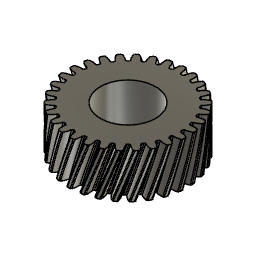
Helical Gear (Autodesk Fusion 360 design; units mm, degrees)
Autodesk Fusion 360 part; units mm, degrees
sketch "Base" plane through (0, 0, 0) normal (0, 0, 1) x (1, 0, 0)
  line L0 (0, 0) -> (8, 0) construction
  arc A0 (0.3264, 4.7068) -> (0.2135, 5.3108) centre (-1.2536, 4.724) ccw
  arc A1 (0.4834, 4.5997) -> (0.4173, 4.6061) centre (0, 0) ccw
  arc A2 (0.1229, 5.3736) -> (0, 5.375) centre (0, 0) ccw
  arc A3 (0.2135, 5.3108) -> (0.1229, 5.3736) centre (0.1206, 5.2736) ccw
  arc A4 (0.3264, 4.7068) -> (0.4173, 4.6061) centre (0.4264, 4.7057) ccw
  arc A5 (0, 5.375) -> (-0.1229, 5.3736) centre (0, 0) ccw
  arc A6 (-0.1229, 5.3736) -> (-0.2135, 5.3108) centre (-0.1206, 5.2736) ccw
  arc A7 (-0.2135, 5.3108) -> (-0.3264, 4.7068) centre (1.2536, 4.724) ccw
  arc A8 (-0.4173, 4.6061) -> (-0.3264, 4.7068) centre (-0.4264, 4.7057) ccw
  arc A9 (-0.4173, 4.6061) -> (-0.4834, 4.5997) centre (0, 0) ccw
  arc A10 (-1.1175, 5.2575) -> (-1.2375, 5.2306) centre (0, 0) ccw
  arc A11 (-0.997, 5.2817) -> (-1.1175, 5.2575) centre (0, 0) ccw
  arc A12 (-1.3659, 4.4187) -> (-1.2978, 4.5361) centre (-1.3954, 4.5142) ccw
  arc A13 (-0.6594, 4.6718) -> (-0.5494, 4.5922) centre (-0.5613, 4.6915) ccw
  arc A14 (-0.8954, 5.2391) -> (-0.997, 5.2817) centre (-0.9785, 5.1835) ccw
  arc A15 (-0.4834, 4.5997) -> (-0.5494, 4.5922) centre (0, 0) ccw
  arc A16 (-1.2375, 5.2306) -> (-1.313, 5.1503) centre (-1.2144, 5.1333) ccw
  arc A17 (-1.3659, 4.4187) -> (-1.4292, 4.3986) centre (0, 0) ccw
  arc A18 (-1.313, 5.1503) -> (-1.2978, 4.5361) centre (0.244, 4.8814) ccw
  arc A19 (-0.6594, 4.6718) -> (-0.8954, 5.2391) centre (-2.2084, 4.3601) ccw
  arc A20 (-2.1862, 4.9103) -> (-2.2979, 4.859) centre (0, 0) ccw
  arc A21 (-2.0734, 4.959) -> (-2.1862, 4.9103) centre (0, 0) ccw
  arc A22 (-2.2548, 4.0382) -> (-2.2126, 4.1671) centre (-2.3035, 4.1255) ccw
  arc A23 (-1.6163, 4.4326) -> (-1.4922, 4.3777) centre (-1.5245, 4.4723) ccw
  arc A24 (-1.9651, 4.9384) -> (-2.0734, 4.959) centre (-2.0348, 4.8668) ccw
  arc A25 (-1.4292, 4.3986) -> (-1.4922, 4.3777) centre (0, 0) ccw
  arc A26 (-2.2979, 4.859) -> (-2.3551, 4.7648) centre (-2.2552, 4.7686) ccw
  arc A27 (-2.2548, 4.0382) -> (-2.3125, 4.0054) centre (0, 0) ccw
  arc A28 (-2.3551, 4.7648) -> (-2.2126, 4.1671) centre (-0.7762, 4.8254) ccw
  arc A29 (-1.6163, 4.4326) -> (-1.9651, 4.9384) centre (-3.0666, 3.8057) ccw
  arc A30 (-3.1593, 4.3485) -> (-3.258, 4.2751) centre (0, 0) ccw
  arc A31 (-3.0591, 4.4196) -> (-3.1593, 4.3485) centre (0, 0) ccw
  arc A32 (-3.0451, 3.4811) -> (-3.0306, 3.616) centre (-3.1109, 3.5564) ccw
  arc A33 (-2.5025, 3.9997) -> (-2.3698, 3.9718) centre (-2.421, 4.0576) ccw
  arc A34 (-2.9489, 4.422) -> (-3.0591, 4.4196) centre (-3.0022, 4.3373) ccw
  arc A35 (-2.3125, 4.0054) -> (-2.3698, 3.9718) centre (0, 0) ccw
  arc A36 (-3.258, 4.2751) -> (-3.2943, 4.171) centre (-3.1973, 4.1956) ccw
  arc A37 (-3.0451, 3.4811) -> (-3.0947, 3.437) centre (0, 0) ccw
  arc A38 (-3.2943, 4.171) -> (-3.0306, 3.616) centre (-1.7625, 4.5586) ccw
  arc A39 (-2.5025, 3.9997) -> (-2.9489, 4.422) centre (-3.7908, 3.0849) ccw
  arc A40 (-3.9944, 3.5966) -> (-4.0756, 3.5043) centre (0, 0) ccw
  arc A41 (-3.9111, 3.687) -> (-3.9944, 3.5966) centre (0, 0) ccw
  arc A42 (-3.7023, 2.772) -> (-3.7162, 2.9069) centre (-3.7823, 2.8319) ccw
  arc A43 (-3.2794, 3.392) -> (-3.1438, 3.3923) centre (-3.2117, 3.4656) ccw
  arc A44 (-3.8038, 3.7122) -> (-3.9111, 3.687) centre (-3.8384, 3.6184) ccw
  arc A45 (-3.0947, 3.437) -> (-3.1438, 3.3923) centre (0, 0) ccw
  arc A46 (-4.0756, 3.5043) -> (-4.0895, 3.395) centre (-3.9998, 3.4391) ccw
  arc A47 (-3.7023, 2.772) -> (-3.7417, 2.7185) centre (0, 0) ccw
  arc A48 (-4.0895, 3.395) -> (-3.7162, 2.9069) centre (-2.6718, 4.0925) ccw
  arc A49 (-3.2794, 3.392) -> (-3.8038, 3.7122) centre (-4.3494, 2.2294) ccw
  arc A50 (-4.6549, 2.6875) -> (-4.7151, 2.5804) centre (0, 0) ccw
  arc A51 (-4.5922, 2.7932) -> (-4.6549, 2.6875) centre (0, 0) ccw
  arc A52 (-4.1977, 1.9416) -> (-4.2394, 2.0708) centre (-4.2885, 1.9836) ccw
  arc A53 (-3.913, 2.6361) -> (-3.7804, 2.6645) centre (-3.8621, 2.7221) ccw
  arc A54 (-4.4925, 2.8402) -> (-4.5922, 2.7932) centre (-4.5068, 2.7413) ccw
  arc A55 (-3.7417, 2.7185) -> (-3.7804, 2.6645) centre (0, 0) ccw
  arc A56 (-4.7151, 2.5804) -> (-4.706, 2.4705) centre (-4.6274, 2.5324) ccw
  arc A57 (-4.1977, 1.9416) -> (-4.2251, 1.8812) centre (0, 0) ccw
  arc A58 (-4.706, 2.4705) -> (-4.2394, 2.0708) centre (-3.4643, 3.4476) ccw
  arc A59 (-3.913, 2.6361) -> (-4.4925, 2.8402) centre (-4.7179, 1.2763) ccw
  arc A60 (-5.1119, 1.661) -> (-5.1486, 1.5436) centre (0, 0) ccw
  arc A61 (-5.0726, 1.7774) -> (-5.1119, 1.661) centre (0, 0) ccw
  arc A62 (-4.5097, 1.0264) -> (-4.5773, 1.1441) centre (-4.6072, 1.0486) ccw
  arc A63 (-4.3756, 1.7649) -> (-4.2517, 1.8203) centre (-4.3437, 1.8597) ccw
  arc A64 (-4.9849, 1.8441) -> (-5.0726, 1.7774) centre (-4.9782, 1.7444) ccw
  arc A65 (-4.2251, 1.8812) -> (-4.2517, 1.8203) centre (0, 0) ccw
  arc A66 (-5.1486, 1.5436) -> (-5.1168, 1.4381) centre (-5.0528, 1.5149) ccw
  arc A67 (-4.5097, 1.0264) -> (-4.5239, 0.9616) centre (0, 0) ccw
  arc A68 (-5.1168, 1.4381) -> (-4.5773, 1.1441) centre (-4.1054, 2.652) ccw
  arc A69 (-4.3756, 1.7649) -> (-4.9849, 1.8441) centre (-4.8801, 0.2676) ccw
  arc A70 (-5.3456, 0.5618) -> (-5.357, 0.4395) centre (0, 0) ccw
  arc A71 (-5.3313, 0.6839) -> (-5.3456, 0.5618) centre (0, 0) ccw
  arc A72 (-4.6245, 0.0664) -> (-4.7151, 0.1674) centre (-4.7245, 0.0678) ccw
  arc A73 (-4.6469, 0.8166) -> (-4.5373, 0.8965) centre (-4.6354, 0.9159) ccw
  arc A74 (-5.2594, 0.7674) -> (-5.3313, 0.6839) centre (-5.2321, 0.6712) ccw
  arc A75 (-4.5239, 0.9616) -> (-4.5373, 0.8965) centre (0, 0) ccw
  arc A76 (-5.357, 0.4395) -> (-5.304, 0.3428) centre (-5.2573, 0.4313) ccw
  arc A77 (-4.6245, 0.0664) -> (-4.625, 0) centre (0, 0) ccw
  arc A78 (-5.304, 0.3428) -> (-4.7151, 0.1674) centre (-4.567, 1.7405) ccw
  arc A79 (-4.6469, 0.8166) -> (-5.2594, 0.7674) centre (-4.8291, -0.7529) ccw
  arc A80 (-5.3456, -0.5618) -> (-5.3313, -0.6839) centre (0, 0) ccw
  arc A81 (-5.357, -0.4395) -> (-5.3456, -0.5618) centre (0, 0) ccw
  arc A82 (-4.5373, -0.8965) -> (-4.6469, -0.8166) centre (-4.6354, -0.9159) ccw
  arc A83 (-4.7151, -0.1674) -> (-4.6245, -0.0664) centre (-4.7245, -0.0678) ccw
  arc A84 (-5.304, -0.3428) -> (-5.357, -0.4395) centre (-5.2573, -0.4313) ccw
  arc A85 (-4.625, 0) -> (-4.6245, -0.0664) centre (0, 0) ccw
  arc A86 (-5.3313, -0.6839) -> (-5.2594, -0.7674) centre (-5.2321, -0.6712) ccw
  arc A87 (-4.5373, -0.8965) -> (-4.5239, -0.9616) centre (0, 0) ccw
  arc A88 (-5.2594, -0.7674) -> (-4.6469, -0.8166) centre (-4.8291, 0.7529) ccw
  arc A89 (-4.7151, -0.1674) -> (-5.304, -0.3428) centre (-4.567, -1.7405) ccw
  arc A90 (-5.1119, -1.661) -> (-5.0726, -1.7774) centre (0, 0) ccw
  arc A91 (-5.1486, -1.5436) -> (-5.1119, -1.661) centre (0, 0) ccw
  arc A92 (-4.2517, -1.8203) -> (-4.3756, -1.7649) centre (-4.3437, -1.8597) ccw
  arc A93 (-4.5773, -1.1441) -> (-4.5097, -1.0264) centre (-4.6072, -1.0486) ccw
  arc A94 (-5.1168, -1.4381) -> (-5.1486, -1.5436) centre (-5.0528, -1.5149) ccw
  arc A95 (-4.5239, -0.9616) -> (-4.5097, -1.0264) centre (0, 0) ccw
  arc A96 (-5.0726, -1.7774) -> (-4.9849, -1.8441) centre (-4.9782, -1.7444) ccw
  arc A97 (-4.2517, -1.8203) -> (-4.2251, -1.8812) centre (0, 0) ccw
  arc A98 (-4.9849, -1.8441) -> (-4.3756, -1.7649) centre (-4.8801, -0.2676) ccw
  arc A99 (-4.5773, -1.1441) -> (-5.1168, -1.4381) centre (-4.1054, -2.652) ccw
  arc A100 (-4.6549, -2.6875) -> (-4.5922, -2.7932) centre (0, 0) ccw
  arc A101 (-4.7151, -2.5804) -> (-4.6549, -2.6875) centre (0, 0) ccw
  arc A102 (-3.7804, -2.6645) -> (-3.913, -2.6361) centre (-3.8621, -2.7221) ccw
  arc A103 (-4.2394, -2.0708) -> (-4.1977, -1.9416) centre (-4.2885, -1.9836) ccw
  arc A104 (-4.706, -2.4705) -> (-4.7151, -2.5804) centre (-4.6274, -2.5324) ccw
  arc A105 (-4.2251, -1.8812) -> (-4.1977, -1.9416) centre (0, 0) ccw
  arc A106 (-4.5922, -2.7932) -> (-4.4925, -2.8402) centre (-4.5068, -2.7413) ccw
  arc A107 (-3.7804, -2.6645) -> (-3.7417, -2.7185) centre (0, 0) ccw
  arc A108 (-4.4925, -2.8402) -> (-3.913, -2.6361) centre (-4.7179, -1.2763) ccw
  arc A109 (-4.2394, -2.0708) -> (-4.706, -2.4705) centre (-3.4643, -3.4476) ccw
  arc A110 (-3.9944, -3.5966) -> (-3.9111, -3.687) centre (0, 0) ccw
  arc A111 (-4.0756, -3.5043) -> (-3.9944, -3.5966) centre (0, 0) ccw
  arc A112 (-3.1438, -3.3923) -> (-3.2794, -3.392) centre (-3.2117, -3.4656) ccw
  arc A113 (-3.7162, -2.9069) -> (-3.7023, -2.772) centre (-3.7823, -2.8319) ccw
  arc A114 (-4.0895, -3.395) -> (-4.0756, -3.5043) centre (-3.9998, -3.4391) ccw
  arc A115 (-3.7417, -2.7185) -> (-3.7023, -2.772) centre (0, 0) ccw
  arc A116 (-3.9111, -3.687) -> (-3.8038, -3.7122) centre (-3.8384, -3.6184) ccw
  arc A117 (-3.1438, -3.3923) -> (-3.0947, -3.437) centre (0, 0) ccw
  arc A118 (-3.8038, -3.7122) -> (-3.2794, -3.392) centre (-4.3494, -2.2294) ccw
  arc A119 (-3.7162, -2.9069) -> (-4.0895, -3.395) centre (-2.6718, -4.0925) ccw
  arc A120 (-3.1593, -4.3485) -> (-3.0591, -4.4196) centre (0, 0) ccw
  arc A121 (-3.258, -4.2751) -> (-3.1593, -4.3485) centre (0, 0) ccw
  arc A122 (-2.3698, -3.9718) -> (-2.5025, -3.9997) centre (-2.421, -4.0576) ccw
  arc A123 (-3.0306, -3.616) -> (-3.0451, -3.4811) centre (-3.1109, -3.5564) ccw
  arc A124 (-3.2943, -4.171) -> (-3.258, -4.2751) centre (-3.1973, -4.1956) ccw
  arc A125 (-3.0947, -3.437) -> (-3.0451, -3.4811) centre (0, 0) ccw
  arc A126 (-3.0591, -4.4196) -> (-2.9489, -4.422) centre (-3.0022, -4.3373) ccw
  arc A127 (-2.3698, -3.9718) -> (-2.3125, -4.0054) centre (0, 0) ccw
  arc A128 (-2.9489, -4.422) -> (-2.5025, -3.9997) centre (-3.7908, -3.0849) ccw
  arc A129 (-3.0306, -3.616) -> (-3.2943, -4.171) centre (-1.7625, -4.5586) ccw
  arc A130 (-2.1862, -4.9103) -> (-2.0734, -4.959) centre (0, 0) ccw
  arc A131 (-2.2979, -4.859) -> (-2.1862, -4.9103) centre (0, 0) ccw
  arc A132 (-1.4922, -4.3777) -> (-1.6163, -4.4326) centre (-1.5245, -4.4723) ccw
  arc A133 (-2.2126, -4.1671) -> (-2.2548, -4.0382) centre (-2.3035, -4.1255) ccw
  arc A134 (-2.3551, -4.7648) -> (-2.2979, -4.859) centre (-2.2552, -4.7686) ccw
  arc A135 (-2.3125, -4.0054) -> (-2.2548, -4.0382) centre (0, 0) ccw
  arc A136 (-2.0734, -4.959) -> (-1.9651, -4.9384) centre (-2.0348, -4.8668) ccw
  arc A137 (-1.4922, -4.3777) -> (-1.4292, -4.3986) centre (0, 0) ccw
  arc A138 (-1.9651, -4.9384) -> (-1.6163, -4.4326) centre (-3.0666, -3.8057) ccw
  arc A139 (-2.2126, -4.1671) -> (-2.3551, -4.7648) centre (-0.7762, -4.8254) ccw
  arc A140 (-1.1175, -5.2575) -> (-0.997, -5.2817) centre (0, 0) ccw
  arc A141 (-1.2375, -5.2306) -> (-1.1175, -5.2575) centre (0, 0) ccw
  arc A142 (-0.5494, -4.5922) -> (-0.6594, -4.6718) centre (-0.5613, -4.6915) ccw
  arc A143 (-1.2978, -4.5361) -> (-1.3659, -4.4187) centre (-1.3954, -4.5142) ccw
  arc A144 (-1.313, -5.1503) -> (-1.2375, -5.2306) centre (-1.2144, -5.1333) ccw
  arc A145 (-1.4292, -4.3986) -> (-1.3659, -4.4187) centre (0, 0) ccw
  arc A146 (-0.997, -5.2817) -> (-0.8954, -5.2391) centre (-0.9785, -5.1835) ccw
  arc A147 (-0.5494, -4.5922) -> (-0.4834, -4.5997) centre (0, 0) ccw
  arc A148 (-0.8954, -5.2391) -> (-0.6594, -4.6718) centre (-2.2084, -4.3601) ccw
  arc A149 (-1.2978, -4.5361) -> (-1.313, -5.1503) centre (0.244, -4.8814) ccw
  arc A150 (0, -5.375) -> (0.1229, -5.3736) centre (0, 0) ccw
  arc A151 (-0.1229, -5.3736) -> (0, -5.375) centre (0, 0) ccw
  arc A152 (0.4173, -4.6061) -> (0.3264, -4.7068) centre (0.4264, -4.7057) ccw
  arc A153 (-0.3264, -4.7068) -> (-0.4173, -4.6061) centre (-0.4264, -4.7057) ccw
  arc A154 (-0.2135, -5.3108) -> (-0.1229, -5.3736) centre (-0.1206, -5.2736) ccw
  arc A155 (-0.4834, -4.5997) -> (-0.4173, -4.6061) centre (0, 0) ccw
  arc A156 (0.1229, -5.3736) -> (0.2135, -5.3108) centre (0.1206, -5.2736) ccw
  arc A157 (0.4173, -4.6061) -> (0.4834, -4.5997) centre (0, 0) ccw
  arc A158 (0.2135, -5.3108) -> (0.3264, -4.7068) centre (-1.2536, -4.724) ccw
  arc A159 (-0.3264, -4.7068) -> (-0.2135, -5.3108) centre (1.2536, -4.724) ccw
  arc A160 (1.1175, -5.2575) -> (1.2375, -5.2306) centre (0, 0) ccw
  arc A161 (0.997, -5.2817) -> (1.1175, -5.2575) centre (0, 0) ccw
  arc A162 (1.3659, -4.4187) -> (1.2978, -4.5361) centre (1.3954, -4.5142) ccw
  arc A163 (0.6594, -4.6718) -> (0.5494, -4.5922) centre (0.5613, -4.6915) ccw
  arc A164 (0.8954, -5.2391) -> (0.997, -5.2817) centre (0.9785, -5.1835) ccw
  arc A165 (0.4834, -4.5997) -> (0.5494, -4.5922) centre (0, 0) ccw
  arc A166 (1.2375, -5.2306) -> (1.313, -5.1503) centre (1.2144, -5.1333) ccw
  arc A167 (1.3659, -4.4187) -> (1.4292, -4.3986) centre (0, 0) ccw
  arc A168 (1.313, -5.1503) -> (1.2978, -4.5361) centre (-0.244, -4.8814) ccw
  arc A169 (0.6594, -4.6718) -> (0.8954, -5.2391) centre (2.2084, -4.3601) ccw
  arc A170 (2.1862, -4.9103) -> (2.2979, -4.859) centre (0, 0) ccw
  arc A171 (2.0734, -4.959) -> (2.1862, -4.9103) centre (0, 0) ccw
  arc A172 (2.2548, -4.0382) -> (2.2126, -4.1671) centre (2.3035, -4.1255) ccw
  arc A173 (1.6163, -4.4326) -> (1.4922, -4.3777) centre (1.5245, -4.4723) ccw
  arc A174 (1.9651, -4.9384) -> (2.0734, -4.959) centre (2.0348, -4.8668) ccw
  arc A175 (1.4292, -4.3986) -> (1.4922, -4.3777) centre (0, 0) ccw
  arc A176 (2.2979, -4.859) -> (2.3551, -4.7648) centre (2.2552, -4.7686) ccw
  arc A177 (2.2548, -4.0382) -> (2.3125, -4.0054) centre (0, 0) ccw
  arc A178 (2.3551, -4.7648) -> (2.2126, -4.1671) centre (0.7762, -4.8254) ccw
  arc A179 (1.6163, -4.4326) -> (1.9651, -4.9384) centre (3.0666, -3.8057) ccw
  arc A180 (3.1593, -4.3485) -> (3.258, -4.2751) centre (0, 0) ccw
  arc A181 (3.0591, -4.4196) -> (3.1593, -4.3485) centre (0, 0) ccw
  arc A182 (3.0451, -3.4811) -> (3.0306, -3.616) centre (3.1109, -3.5564) ccw
  arc A183 (2.5025, -3.9997) -> (2.3698, -3.9718) centre (2.421, -4.0576) ccw
  arc A184 (2.9489, -4.422) -> (3.0591, -4.4196) centre (3.0022, -4.3373) ccw
  arc A185 (2.3125, -4.0054) -> (2.3698, -3.9718) centre (0, 0) ccw
  arc A186 (3.258, -4.2751) -> (3.2943, -4.171) centre (3.1973, -4.1956) ccw
  arc A187 (3.0451, -3.4811) -> (3.0947, -3.437) centre (0, 0) ccw
  arc A188 (3.2943, -4.171) -> (3.0306, -3.616) centre (1.7625, -4.5586) ccw
  arc A189 (2.5025, -3.9997) -> (2.9489, -4.422) centre (3.7908, -3.0849) ccw
  arc A190 (3.9944, -3.5966) -> (4.0756, -3.5043) centre (0, 0) ccw
  arc A191 (3.9111, -3.687) -> (3.9944, -3.5966) centre (0, 0) ccw
  arc A192 (3.7023, -2.772) -> (3.7162, -2.9069) centre (3.7823, -2.8319) ccw
  arc A193 (3.2794, -3.392) -> (3.1438, -3.3923) centre (3.2117, -3.4656) ccw
  arc A194 (3.8038, -3.7122) -> (3.9111, -3.687) centre (3.8384, -3.6184) ccw
  arc A195 (3.0947, -3.437) -> (3.1438, -3.3923) centre (0, 0) ccw
  arc A196 (4.0756, -3.5043) -> (4.0895, -3.395) centre (3.9998, -3.4391) ccw
  arc A197 (3.7023, -2.772) -> (3.7417, -2.7185) centre (0, 0) ccw
  arc A198 (4.0895, -3.395) -> (3.7162, -2.9069) centre (2.6718, -4.0925) ccw
  arc A199 (3.2794, -3.392) -> (3.8038, -3.7122) centre (4.3494, -2.2294) ccw
  arc A200 (4.6549, -2.6875) -> (4.7151, -2.5804) centre (0, 0) ccw
  arc A201 (4.5922, -2.7932) -> (4.6549, -2.6875) centre (0, 0) ccw
  arc A202 (4.1977, -1.9416) -> (4.2394, -2.0708) centre (4.2885, -1.9836) ccw
  arc A203 (3.913, -2.6361) -> (3.7804, -2.6645) centre (3.8621, -2.7221) ccw
  arc A204 (4.4925, -2.8402) -> (4.5922, -2.7932) centre (4.5068, -2.7413) ccw
  arc A205 (3.7417, -2.7185) -> (3.7804, -2.6645) centre (0, 0) ccw
  arc A206 (4.7151, -2.5804) -> (4.706, -2.4705) centre (4.6274, -2.5324) ccw
  arc A207 (4.1977, -1.9416) -> (4.2251, -1.8812) centre (0, 0) ccw
  arc A208 (4.706, -2.4705) -> (4.2394, -2.0708) centre (3.4643, -3.4476) ccw
  arc A209 (3.913, -2.6361) -> (4.4925, -2.8402) centre (4.7179, -1.2763) ccw
  arc A210 (5.1119, -1.661) -> (5.1486, -1.5436) centre (0, 0) ccw
  arc A211 (5.0726, -1.7774) -> (5.1119, -1.661) centre (0, 0) ccw
  arc A212 (4.5097, -1.0264) -> (4.5773, -1.1441) centre (4.6072, -1.0486) ccw
  arc A213 (4.3756, -1.7649) -> (4.2517, -1.8203) centre (4.3437, -1.8597) ccw
  arc A214 (4.9849, -1.8441) -> (5.0726, -1.7774) centre (4.9782, -1.7444) ccw
  arc A215 (4.2251, -1.8812) -> (4.2517, -1.8203) centre (0, 0) ccw
  arc A216 (5.1486, -1.5436) -> (5.1168, -1.4381) centre (5.0528, -1.5149) ccw
  arc A217 (4.5097, -1.0264) -> (4.5239, -0.9616) centre (0, 0) ccw
  arc A218 (5.1168, -1.4381) -> (4.5773, -1.1441) centre (4.1054, -2.652) ccw
  arc A219 (4.3756, -1.7649) -> (4.9849, -1.8441) centre (4.8801, -0.2676) ccw
  arc A220 (5.3456, -0.5618) -> (5.357, -0.4395) centre (0, 0) ccw
  arc A221 (5.3313, -0.6839) -> (5.3456, -0.5618) centre (0, 0) ccw
  arc A222 (4.6245, -0.0664) -> (4.7151, -0.1674) centre (4.7245, -0.0678) ccw
  arc A223 (4.6469, -0.8166) -> (4.5373, -0.8965) centre (4.6354, -0.9159) ccw
  arc A224 (5.2594, -0.7674) -> (5.3313, -0.6839) centre (5.2321, -0.6712) ccw
  arc A225 (4.5239, -0.9616) -> (4.5373, -0.8965) centre (0, 0) ccw
  arc A226 (5.357, -0.4395) -> (5.304, -0.3428) centre (5.2573, -0.4313) ccw
  arc A227 (4.6245, -0.0664) -> (4.625, 0) centre (0, 0) ccw
  arc A228 (5.304, -0.3428) -> (4.7151, -0.1674) centre (4.567, -1.7405) ccw
  arc A229 (4.6469, -0.8166) -> (5.2594, -0.7674) centre (4.8291, 0.7529) ccw
  arc A230 (5.3456, 0.5618) -> (5.3313, 0.6839) centre (0, 0) ccw
  arc A231 (5.357, 0.4395) -> (5.3456, 0.5618) centre (0, 0) ccw
  arc A232 (4.5373, 0.8965) -> (4.6469, 0.8166) centre (4.6354, 0.9159) ccw
  arc A233 (4.7151, 0.1674) -> (4.6245, 0.0664) centre (4.7245, 0.0678) ccw
  arc A234 (5.304, 0.3428) -> (5.357, 0.4395) centre (5.2573, 0.4313) ccw
  arc A235 (4.625, 0) -> (4.6245, 0.0664) centre (0, 0) ccw
  arc A236 (5.3313, 0.6839) -> (5.2594, 0.7674) centre (5.2321, 0.6712) ccw
  arc A237 (4.5373, 0.8965) -> (4.5239, 0.9616) centre (0, 0) ccw
  arc A238 (5.2594, 0.7674) -> (4.6469, 0.8166) centre (4.8291, -0.7529) ccw
  arc A239 (4.7151, 0.1674) -> (5.304, 0.3428) centre (4.567, 1.7405) ccw
  arc A240 (5.1119, 1.661) -> (5.0726, 1.7774) centre (0, 0) ccw
  arc A241 (5.1486, 1.5436) -> (5.1119, 1.661) centre (0, 0) ccw
  arc A242 (4.2517, 1.8203) -> (4.3756, 1.7649) centre (4.3437, 1.8597) ccw
  arc A243 (4.5773, 1.1441) -> (4.5097, 1.0264) centre (4.6072, 1.0486) ccw
  arc A244 (5.1168, 1.4381) -> (5.1486, 1.5436) centre (5.0528, 1.5149) ccw
  arc A245 (4.5239, 0.9616) -> (4.5097, 1.0264) centre (0, 0) ccw
  arc A246 (5.0726, 1.7774) -> (4.9849, 1.8441) centre (4.9782, 1.7444) ccw
  arc A247 (4.2517, 1.8203) -> (4.2251, 1.8812) centre (0, 0) ccw
  arc A248 (4.9849, 1.8441) -> (4.3756, 1.7649) centre (4.8801, 0.2676) ccw
  arc A249 (4.5773, 1.1441) -> (5.1168, 1.4381) centre (4.1054, 2.652) ccw
  arc A250 (4.6549, 2.6875) -> (4.5922, 2.7932) centre (0, 0) ccw
  arc A251 (4.7151, 2.5804) -> (4.6549, 2.6875) centre (0, 0) ccw
  arc A252 (3.7804, 2.6645) -> (3.913, 2.6361) centre (3.8621, 2.7221) ccw
  arc A253 (4.2394, 2.0708) -> (4.1977, 1.9416) centre (4.2885, 1.9836) ccw
  arc A254 (4.706, 2.4705) -> (4.7151, 2.5804) centre (4.6274, 2.5324) ccw
  arc A255 (4.2251, 1.8812) -> (4.1977, 1.9416) centre (0, 0) ccw
  arc A256 (4.5922, 2.7932) -> (4.4925, 2.8402) centre (4.5068, 2.7413) ccw
  arc A257 (3.7804, 2.6645) -> (3.7417, 2.7185) centre (0, 0) ccw
  arc A258 (4.4925, 2.8402) -> (3.913, 2.6361) centre (4.7179, 1.2763) ccw
  arc A259 (4.2394, 2.0708) -> (4.706, 2.4705) centre (3.4643, 3.4476) ccw
  arc A260 (3.9944, 3.5966) -> (3.9111, 3.687) centre (0, 0) ccw
  arc A261 (4.0756, 3.5043) -> (3.9944, 3.5966) centre (0, 0) ccw
  arc A262 (3.1438, 3.3923) -> (3.2794, 3.392) centre (3.2117, 3.4656) ccw
  arc A263 (3.7162, 2.9069) -> (3.7023, 2.772) centre (3.7823, 2.8319) ccw
  arc A264 (4.0895, 3.395) -> (4.0756, 3.5043) centre (3.9998, 3.4391) ccw
  arc A265 (3.7417, 2.7185) -> (3.7023, 2.772) centre (0, 0) ccw
  arc A266 (3.9111, 3.687) -> (3.8038, 3.7122) centre (3.8384, 3.6184) ccw
  arc A267 (3.1438, 3.3923) -> (3.0947, 3.437) centre (0, 0) ccw
  arc A268 (3.8038, 3.7122) -> (3.2794, 3.392) centre (4.3494, 2.2294) ccw
  arc A269 (3.7162, 2.9069) -> (4.0895, 3.395) centre (2.6718, 4.0925) ccw
  arc A270 (3.1593, 4.3485) -> (3.0591, 4.4196) centre (0, 0) ccw
  arc A271 (3.258, 4.2751) -> (3.1593, 4.3485) centre (0, 0) ccw
  arc A272 (2.3698, 3.9718) -> (2.5025, 3.9997) centre (2.421, 4.0576) ccw
  arc A273 (3.0306, 3.616) -> (3.0451, 3.4811) centre (3.1109, 3.5564) ccw
  arc A274 (3.2943, 4.171) -> (3.258, 4.2751) centre (3.1973, 4.1956) ccw
  arc A275 (3.0947, 3.437) -> (3.0451, 3.4811) centre (0, 0) ccw
  arc A276 (3.0591, 4.4196) -> (2.9489, 4.422) centre (3.0022, 4.3373) ccw
  arc A277 (2.3698, 3.9718) -> (2.3125, 4.0054) centre (0, 0) ccw
  arc A278 (2.9489, 4.422) -> (2.5025, 3.9997) centre (3.7908, 3.0849) ccw
  arc A279 (3.0306, 3.616) -> (3.2943, 4.171) centre (1.7625, 4.5586) ccw
  arc A280 (2.1862, 4.9103) -> (2.0734, 4.959) centre (0, 0) ccw
  arc A281 (2.2979, 4.859) -> (2.1862, 4.9103) centre (0, 0) ccw
  arc A282 (1.4922, 4.3777) -> (1.6163, 4.4326) centre (1.5245, 4.4723) ccw
  arc A283 (2.2126, 4.1671) -> (2.2548, 4.0382) centre (2.3035, 4.1255) ccw
  arc A284 (2.3551, 4.7648) -> (2.2979, 4.859) centre (2.2552, 4.7686) ccw
  arc A285 (2.3125, 4.0054) -> (2.2548, 4.0382) centre (0, 0) ccw
  arc A286 (2.0734, 4.959) -> (1.9651, 4.9384) centre (2.0348, 4.8668) ccw
  arc A287 (1.4922, 4.3777) -> (1.4292, 4.3986) centre (0, 0) ccw
  arc A288 (1.9651, 4.9384) -> (1.6163, 4.4326) centre (3.0666, 3.8057) ccw
  arc A289 (2.2126, 4.1671) -> (2.3551, 4.7648) centre (0.7762, 4.8254) ccw
  arc A290 (1.1175, 5.2575) -> (0.997, 5.2817) centre (0, 0) ccw
  arc A291 (1.2375, 5.2306) -> (1.1175, 5.2575) centre (0, 0) ccw
  arc A292 (0.5494, 4.5922) -> (0.6594, 4.6718) centre (0.5613, 4.6915) ccw
  arc A293 (1.2978, 4.5361) -> (1.3659, 4.4187) centre (1.3954, 4.5142) ccw
  arc A294 (1.313, 5.1503) -> (1.2375, 5.2306) centre (1.2144, 5.1333) ccw
  arc A295 (1.4292, 4.3986) -> (1.3659, 4.4187) centre (0, 0) ccw
  arc A296 (0.997, 5.2817) -> (0.8954, 5.2391) centre (0.9785, 5.1835) ccw
  arc A297 (0.5494, 4.5922) -> (0.4834, 4.5997) centre (0, 0) ccw
  arc A298 (0.8954, 5.2391) -> (0.6594, 4.6718) centre (2.2084, 4.3601) ccw
  arc A299 (1.2978, 4.5361) -> (1.313, 5.1503) centre (-0.244, 4.8814) ccw
  dimension "d7" = 0.1
  dimension "d8" = 0.1
  dimension "d10" = 360
  constraint coincident L0.start A1.centre
  constraint tangent A0 A3
  constraint tangent A2 A3
  constraint tangent A0 A4
  constraint tangent A1 A4
  measures "d7" radius of A3
  measures "d8" radius of A4
sketch "Path" plane through (0, 0, 0) normal (1, 0, 0) x (0, 1, 0)
  line L0 (0, 0) -> (0, 4)
  dimension "d11" = 4
  constraint coincident L0.start origin
  constraint vertical L0
  measures "d11" distance of L0.start L0.end
sweep "Sweep1" add twist angle 15 profiles "Base" path "Path" along L0 section 1
sketch "Cut" plane through (0, 0, 4) normal (0, 0, 1) x (-1, 0, 0)
  arc A0 (-0.3083, -4.6147) -> (-0.1757, -4.6217) centre (0, 0) ccw
  arc A1 (-0.0796, -4.7174) -> (-0.1757, -4.6217) centre (-0.1795, -4.7216) ccw
  arc A2 (-0.0796, -4.7174) -> (0.0648, -5.3147) centre (1.4991, -4.6519) ccw
  arc A3 (0.0648, -5.3147) -> (0.1585, -5.3727) centre (0.1555, -5.2727) ccw
  arc A4 (0.1585, -5.3727) -> (0.404, -5.3598) centre (0, 0) ccw
  arc A5 (0.404, -5.3598) -> (0.4911, -5.2923) centre (0.3965, -5.2601) ccw
  arc A6 (0.4911, -5.2923) -> (0.5723, -4.6833) centre (-1.0046, -4.7831) ccw
  arc A7 (0.6578, -4.578) -> (0.5723, -4.6833) centre (0.6721, -4.677) ccw
  arc A8 (0.6578, -4.578) -> (0.789, -4.5572) centre (0, 0) ccw
  arc A9 (0.903, -4.6309) -> (0.789, -4.5572) centre (0.8061, -4.6557) ccw
  arc A10 (0.903, -4.6309) -> (1.1683, -5.185) centre (2.4335, -4.2385) ccw
  arc A11 (1.1683, -5.185) -> (1.2721, -5.2223) centre (1.2484, -5.1251) ccw
  arc A12 (1.2721, -5.2223) -> (1.5095, -5.1587) centre (0, 0) ccw
  arc A13 (1.5095, -5.1587) -> (1.5807, -5.0746) centre (1.4814, -5.0627) ccw
  arc A14 (1.5807, -5.0746) -> (1.5335, -4.462) centre (0.0118, -4.8874) ccw
  arc A15 (1.5953, -4.3412) -> (1.5335, -4.462) centre (1.6298, -4.435) ccw
  arc A16 (1.5953, -4.3412) -> (1.7193, -4.2936) centre (0, 0) ccw
  arc A17 (1.846, -4.342) -> (1.7193, -4.2936) centre (1.7565, -4.3864) ccw
  arc A18 (1.846, -4.342) -> (2.2208, -4.8288) centre (3.2616, -3.64) ccw
  arc A19 (2.2208, -4.8288) -> (2.3301, -4.8437) centre (2.2867, -4.7536) ccw
  arc A20 (2.3301, -4.8437) -> (2.5491, -4.7321) centre (0, 0) ccw
  arc A21 (2.5491, -4.7321) -> (2.6012, -4.635) centre (2.5016, -4.6441) ccw
  arc A22 (2.6012, -4.635) -> (2.4277, -4.0456) centre (1.0277, -4.7782) ccw
  arc A23 (2.463, -3.9146) -> (2.4277, -4.0456) centre (2.5163, -3.9993) ccw
  arc A24 (2.463, -3.9146) -> (2.5744, -3.8423) centre (0, 0) ccw
  arc A25 (2.7084, -3.8633) -> (2.5744, -3.8423) centre (2.6301, -3.9254) ccw
  arc A26 (2.7084, -3.8633) -> (3.1763, -4.2616) centre (3.9471, -2.8823) ccw
  arc A27 (3.1763, -4.2616) -> (3.2862, -4.2534) centre (3.2251, -4.1743) ccw
  arc A28 (3.2862, -4.2534) -> (3.4772, -4.0987) centre (0, 0) ccw
  arc A29 (3.4772, -4.0987) -> (3.5081, -3.9929) centre (3.4125, -4.0225) ccw
  arc A30 (3.5081, -3.9929) -> (3.2157, -3.4525) centre (1.9987, -4.4601) ccw
  arc A31 (3.2231, -3.317) -> (3.2157, -3.4525) centre (3.2928, -3.3887) ccw
  arc A32 (3.2231, -3.317) -> (3.317, -3.2231) centre (0, 0) ccw
  arc A33 (3.4525, -3.2157) -> (3.317, -3.2231) centre (3.3887, -3.2928) ccw
  arc A34 (3.4525, -3.2157) -> (3.9929, -3.5081) centre (4.4601, -1.9987) ccw
  arc A35 (3.9929, -3.5081) -> (4.0987, -3.4772) centre (4.0225, -3.4125) ccw
  arc A36 (4.0987, -3.4772) -> (4.2534, -3.2862) centre (0, 0) ccw
  arc A37 (4.2534, -3.2862) -> (4.2616, -3.1763) centre (4.1743, -3.2251) ccw
  arc A38 (4.2616, -3.1763) -> (3.8633, -2.7084) centre (2.8823, -3.9471) ccw
  arc A39 (3.8423, -2.5744) -> (3.8633, -2.7084) centre (3.9254, -2.6301) ccw
  arc A40 (3.8423, -2.5744) -> (3.9146, -2.463) centre (0, 0) ccw
  arc A41 (4.0456, -2.4277) -> (3.9146, -2.463) centre (3.9993, -2.5163) ccw
  arc A42 (4.0456, -2.4277) -> (4.635, -2.6012) centre (4.7782, -1.0277) ccw
  arc A43 (4.635, -2.6012) -> (4.7321, -2.5491) centre (4.6441, -2.5016) ccw
  arc A44 (4.7321, -2.5491) -> (4.8437, -2.3301) centre (0, 0) ccw
  arc A45 (4.8437, -2.3301) -> (4.8288, -2.2208) centre (4.7536, -2.2867) ccw
  arc A46 (4.8288, -2.2208) -> (4.342, -1.846) centre (3.64, -3.2616) ccw
  arc A47 (4.2936, -1.7193) -> (4.342, -1.846) centre (4.3864, -1.7565) ccw
  arc A48 (4.2936, -1.7193) -> (4.3412, -1.5953) centre (0, 0) ccw
  arc A49 (4.462, -1.5335) -> (4.3412, -1.5953) centre (4.435, -1.6298) ccw
  arc A50 (4.462, -1.5335) -> (5.0746, -1.5807) centre (4.8874, -0.0118) ccw
  arc A51 (5.0746, -1.5807) -> (5.1587, -1.5095) centre (5.0627, -1.4814) ccw
  arc A52 (5.1587, -1.5095) -> (5.2223, -1.2721) centre (0, 0) ccw
  arc A53 (5.2223, -1.2721) -> (5.185, -1.1683) centre (5.1251, -1.2484) ccw
  arc A54 (5.185, -1.1683) -> (4.6309, -0.903) centre (4.2385, -2.4335) ccw
  arc A55 (4.5572, -0.789) -> (4.6309, -0.903) centre (4.6557, -0.8061) ccw
  arc A56 (4.5572, -0.789) -> (4.578, -0.6578) centre (0, 0) ccw
  arc A57 (4.6833, -0.5723) -> (4.578, -0.6578) centre (4.677, -0.6721) ccw
  arc A58 (4.6833, -0.5723) -> (5.2923, -0.4911) centre (4.7831, 1.0046) ccw
  arc A59 (5.2923, -0.4911) -> (5.3598, -0.404) centre (5.2601, -0.3965) ccw
  arc A60 (5.3598, -0.404) -> (5.3727, -0.1585) centre (0, 0) ccw
  arc A61 (5.3727, -0.1585) -> (5.3147, -0.0648) centre (5.2727, -0.1555) ccw
  arc A62 (5.3147, -0.0648) -> (4.7174, 0.0796) centre (4.6519, -1.4991) ccw
  arc A63 (4.6217, 0.1757) -> (4.7174, 0.0796) centre (4.7216, 0.1795) ccw
  arc A64 (4.6217, 0.1757) -> (4.6147, 0.3083) centre (0, 0) ccw
  arc A65 (4.6999, 0.4139) -> (4.6147, 0.3083) centre (4.7145, 0.315) ccw
  arc A66 (4.6999, 0.4139) -> (5.2788, 0.6199) centre (4.4697, 1.9771) ccw
  arc A67 (5.2788, 0.6199) -> (5.3267, 0.7192) centre (5.2276, 0.7058) ccw
  arc A68 (5.3267, 0.7192) -> (5.2882, 0.962) centre (0, 0) ccw
  arc A69 (5.2882, 0.962) -> (5.212, 1.0416) centre (5.1898, 0.9441) ccw
  arc A70 (5.212, 1.0416) -> (4.5978, 1.0587) centre (4.8619, -0.4992) ccw
  arc A71 (4.4841, 1.1328) -> (4.5978, 1.0587) centre (4.5811, 1.1573) ccw
  arc A72 (4.4841, 1.1328) -> (4.4498, 1.2611) centre (0, 0) ccw
  arc A73 (4.5111, 1.3821) -> (4.4498, 1.2611) centre (4.546, 1.2883) ccw
  arc A74 (4.5111, 1.3821) -> (5.0345, 1.7039) centre (3.9609, 2.8632) ccw
  arc A75 (5.0345, 1.7039) -> (5.0607, 1.811) centre (4.9666, 1.7773) ccw
  arc A76 (5.0607, 1.811) -> (4.9726, 2.0405) centre (0, 0) ccw
  arc A77 (4.9726, 2.0405) -> (4.8815, 2.1025) centre (4.8801, 2.0025) ccw
  arc A78 (4.8815, 2.1025) -> (4.2772, 1.9915) centre (4.8594, 0.5226) ccw
  arc A79 (4.1506, 2.0403) -> (4.2772, 1.9915) centre (4.2404, 2.0844) ccw
  arc A80 (4.1506, 2.0403) -> (4.0903, 2.1587) centre (0, 0) ccw
  arc A81 (4.1252, 2.2898) -> (4.0903, 2.1587) centre (4.1788, 2.2053) ccw
  arc A82 (4.1252, 2.2898) -> (4.5702, 2.7134) centre (3.2791, 3.6242) ccw
  arc A83 (4.5702, 2.7134) -> (4.5736, 2.8236) centre (4.4885, 2.7711) ccw
  arc A84 (4.5736, 2.8236) -> (4.4397, 3.0297) centre (0, 0) ccw
  arc A85 (4.4397, 3.0297) -> (4.3377, 3.0715) centre (4.3571, 2.9734) ccw
  arc A86 (4.3377, 3.0715) -> (3.7697, 2.8372) centre (4.6446, 1.5215) ccw
  arc A87 (3.6357, 2.8587) -> (3.7697, 2.8372) centre (3.7143, 2.9205) ccw
  arc A88 (3.6357, 2.8587) -> (3.5521, 2.9619) centre (0, 0) ccw
  arc A89 (3.559, 3.0974) -> (3.5521, 2.9619) centre (3.6289, 3.026) ccw
  arc A90 (3.559, 3.0974) -> (3.9062, 3.6043) centre (2.4539, 4.2268) ccw
  arc A91 (3.9062, 3.6043) -> (3.8866, 3.7128) centre (3.8143, 3.6437) ccw
  arc A92 (3.8866, 3.7128) -> (3.7128, 3.8866) centre (0, 0) ccw
  arc A93 (3.7128, 3.8866) -> (3.6043, 3.9062) centre (3.6437, 3.8143) ccw
  arc A94 (3.6043, 3.9062) -> (3.0974, 3.559) centre (4.2268, 2.4539) ccw
  arc A95 (2.9619, 3.5521) -> (3.0974, 3.559) centre (3.026, 3.6289) ccw
  arc A96 (2.9619, 3.5521) -> (2.8587, 3.6357) centre (0, 0) ccw
  arc A97 (2.8372, 3.7697) -> (2.8587, 3.6357) centre (2.9205, 3.7143) ccw
  arc A98 (2.8372, 3.7697) -> (3.0715, 4.3377) centre (1.5215, 4.6446) ccw
  arc A99 (3.0715, 4.3377) -> (3.0297, 4.4397) centre (2.9734, 4.3571) ccw
  arc A100 (3.0297, 4.4397) -> (2.8236, 4.5736) centre (0, 0) ccw
  arc A101 (2.8236, 4.5736) -> (2.7134, 4.5702) centre (2.7711, 4.4885) ccw
  arc A102 (2.7134, 4.5702) -> (2.2898, 4.1252) centre (3.6242, 3.2791) ccw
  arc A103 (2.1587, 4.0903) -> (2.2898, 4.1252) centre (2.2053, 4.1788) ccw
  arc A104 (2.1587, 4.0903) -> (2.0403, 4.1506) centre (0, 0) ccw
  arc A105 (1.9915, 4.2772) -> (2.0403, 4.1506) centre (2.0844, 4.2404) ccw
  arc A106 (1.9915, 4.2772) -> (2.1025, 4.8815) centre (0.5226, 4.8594) ccw
  arc A107 (2.1025, 4.8815) -> (2.0405, 4.9726) centre (2.0025, 4.8801) ccw
  arc A108 (2.0405, 4.9726) -> (1.811, 5.0607) centre (0, 0) ccw
  arc A109 (1.811, 5.0607) -> (1.7039, 5.0345) centre (1.7773, 4.9666) ccw
  arc A110 (1.7039, 5.0345) -> (1.3821, 4.5111) centre (2.8632, 3.9609) ccw
  arc A111 (1.2611, 4.4498) -> (1.3821, 4.5111) centre (1.2883, 4.546) ccw
  arc A112 (1.2611, 4.4498) -> (1.1328, 4.4841) centre (0, 0) ccw
  arc A113 (1.0587, 4.5978) -> (1.1328, 4.4841) centre (1.1573, 4.5811) ccw
  arc A114 (1.0587, 4.5978) -> (1.0416, 5.212) centre (-0.4992, 4.8619) ccw
  arc A115 (1.0416, 5.212) -> (0.962, 5.2882) centre (0.9441, 5.1898) ccw
  arc A116 (0.962, 5.2882) -> (0.7192, 5.3267) centre (0, 0) ccw
  arc A117 (0.7192, 5.3267) -> (0.6199, 5.2788) centre (0.7058, 5.2276) ccw
  arc A118 (0.6199, 5.2788) -> (0.4139, 4.6999) centre (1.9771, 4.4697) ccw
  arc A119 (0.3083, 4.6147) -> (0.4139, 4.6999) centre (0.315, 4.7145) ccw
  arc A120 (0.3083, 4.6147) -> (0.1757, 4.6217) centre (0, 0) ccw
  arc A121 (0.0796, 4.7174) -> (0.1757, 4.6217) centre (0.1795, 4.7216) ccw
  arc A122 (0.0796, 4.7174) -> (-0.0648, 5.3147) centre (-1.4991, 4.6519) ccw
  arc A123 (-0.0648, 5.3147) -> (-0.1585, 5.3727) centre (-0.1555, 5.2727) ccw
  arc A124 (-0.1585, 5.3727) -> (-0.404, 5.3598) centre (0, 0) ccw
  arc A125 (-0.404, 5.3598) -> (-0.4911, 5.2923) centre (-0.3965, 5.2601) ccw
  arc A126 (-0.4911, 5.2923) -> (-0.5723, 4.6833) centre (1.0046, 4.7831) ccw
  arc A127 (-0.6578, 4.578) -> (-0.5723, 4.6833) centre (-0.6721, 4.677) ccw
  arc A128 (-0.6578, 4.578) -> (-0.789, 4.5572) centre (0, 0) ccw
  arc A129 (-0.903, 4.6309) -> (-0.789, 4.5572) centre (-0.8061, 4.6557) ccw
  arc A130 (-0.903, 4.6309) -> (-1.1683, 5.185) centre (-2.4335, 4.2385) ccw
  arc A131 (-1.1683, 5.185) -> (-1.2721, 5.2223) centre (-1.2484, 5.1251) ccw
  arc A132 (-1.2721, 5.2223) -> (-1.5095, 5.1587) centre (0, 0) ccw
  arc A133 (-1.5095, 5.1587) -> (-1.5807, 5.0746) centre (-1.4814, 5.0627) ccw
  arc A134 (-1.5807, 5.0746) -> (-1.5335, 4.462) centre (-0.0118, 4.8874) ccw
  arc A135 (-1.5953, 4.3412) -> (-1.5335, 4.462) centre (-1.6298, 4.435) ccw
  arc A136 (-1.5953, 4.3412) -> (-1.7193, 4.2936) centre (0, 0) ccw
  arc A137 (-1.846, 4.342) -> (-1.7193, 4.2936) centre (-1.7565, 4.3864) ccw
  arc A138 (-1.846, 4.342) -> (-2.2208, 4.8288) centre (-3.2616, 3.64) ccw
  arc A139 (-2.2208, 4.8288) -> (-2.3301, 4.8437) centre (-2.2867, 4.7536) ccw
  arc A140 (-2.3301, 4.8437) -> (-2.5491, 4.7321) centre (0, 0) ccw
  arc A141 (-2.5491, 4.7321) -> (-2.6012, 4.635) centre (-2.5016, 4.6441) ccw
  arc A142 (-2.6012, 4.635) -> (-2.4277, 4.0456) centre (-1.0277, 4.7782) ccw
  arc A143 (-2.463, 3.9146) -> (-2.4277, 4.0456) centre (-2.5163, 3.9993) ccw
  arc A144 (-2.463, 3.9146) -> (-2.5744, 3.8423) centre (0, 0) ccw
  arc A145 (-2.7084, 3.8633) -> (-2.5744, 3.8423) centre (-2.6301, 3.9254) ccw
  arc A146 (-2.7084, 3.8633) -> (-3.1763, 4.2616) centre (-3.9471, 2.8823) ccw
  arc A147 (-3.1763, 4.2616) -> (-3.2862, 4.2534) centre (-3.2251, 4.1743) ccw
  arc A148 (-3.2862, 4.2534) -> (-3.4772, 4.0987) centre (0, 0) ccw
  arc A149 (-3.4772, 4.0987) -> (-3.5081, 3.9929) centre (-3.4125, 4.0225) ccw
  arc A150 (-3.5081, 3.9929) -> (-3.2157, 3.4525) centre (-1.9987, 4.4601) ccw
  arc A151 (-3.2231, 3.317) -> (-3.2157, 3.4525) centre (-3.2928, 3.3887) ccw
  arc A152 (-3.2231, 3.317) -> (-3.317, 3.2231) centre (0, 0) ccw
  arc A153 (-3.4525, 3.2157) -> (-3.317, 3.2231) centre (-3.3887, 3.2928) ccw
  arc A154 (-3.4525, 3.2157) -> (-3.9929, 3.5081) centre (-4.4601, 1.9987) ccw
  arc A155 (-3.9929, 3.5081) -> (-4.0987, 3.4772) centre (-4.0225, 3.4125) ccw
  arc A156 (-4.0987, 3.4772) -> (-4.2534, 3.2862) centre (0, 0) ccw
  arc A157 (-4.2534, 3.2862) -> (-4.2616, 3.1763) centre (-4.1743, 3.2251) ccw
  arc A158 (-4.2616, 3.1763) -> (-3.8633, 2.7084) centre (-2.8823, 3.9471) ccw
  arc A159 (-3.8423, 2.5744) -> (-3.8633, 2.7084) centre (-3.9254, 2.6301) ccw
  arc A160 (-3.8423, 2.5744) -> (-3.9146, 2.463) centre (0, 0) ccw
  arc A161 (-4.0456, 2.4277) -> (-3.9146, 2.463) centre (-3.9993, 2.5163) ccw
  arc A162 (-4.0456, 2.4277) -> (-4.635, 2.6012) centre (-4.7782, 1.0277) ccw
  arc A163 (-4.635, 2.6012) -> (-4.7321, 2.5491) centre (-4.6441, 2.5016) ccw
  arc A164 (-4.7321, 2.5491) -> (-4.8437, 2.3301) centre (0, 0) ccw
  arc A165 (-4.8437, 2.3301) -> (-4.8288, 2.2208) centre (-4.7536, 2.2867) ccw
  arc A166 (-4.8288, 2.2208) -> (-4.342, 1.846) centre (-3.64, 3.2616) ccw
  arc A167 (-4.2936, 1.7193) -> (-4.342, 1.846) centre (-4.3864, 1.7565) ccw
  arc A168 (-4.2936, 1.7193) -> (-4.3412, 1.5953) centre (0, 0) ccw
  arc A169 (-4.462, 1.5335) -> (-4.3412, 1.5953) centre (-4.435, 1.6298) ccw
  arc A170 (-4.462, 1.5335) -> (-5.0746, 1.5807) centre (-4.8874, 0.0118) ccw
  arc A171 (-5.0746, 1.5807) -> (-5.1587, 1.5095) centre (-5.0627, 1.4814) ccw
  arc A172 (-5.1587, 1.5095) -> (-5.2223, 1.2721) centre (0, 0) ccw
  arc A173 (-5.2223, 1.2721) -> (-5.185, 1.1683) centre (-5.1251, 1.2484) ccw
  arc A174 (-5.185, 1.1683) -> (-4.6309, 0.903) centre (-4.2385, 2.4335) ccw
  arc A175 (-4.5572, 0.789) -> (-4.6309, 0.903) centre (-4.6557, 0.8061) ccw
  arc A176 (-4.5572, 0.789) -> (-4.578, 0.6578) centre (0, 0) ccw
  arc A177 (-4.6833, 0.5723) -> (-4.578, 0.6578) centre (-4.677, 0.6721) ccw
  arc A178 (-4.6833, 0.5723) -> (-5.2923, 0.4911) centre (-4.7831, -1.0046) ccw
  arc A179 (-5.2923, 0.4911) -> (-5.3598, 0.404) centre (-5.2601, 0.3965) ccw
  arc A180 (-5.3598, 0.404) -> (-5.3727, 0.1585) centre (0, 0) ccw
  arc A181 (-5.3727, 0.1585) -> (-5.3147, 0.0648) centre (-5.2727, 0.1555) ccw
  arc A182 (-5.3147, 0.0648) -> (-4.7174, -0.0796) centre (-4.6519, 1.4991) ccw
  arc A183 (-4.6217, -0.1757) -> (-4.7174, -0.0796) centre (-4.7216, -0.1795) ccw
  arc A184 (-4.6217, -0.1757) -> (-4.6147, -0.3083) centre (0, 0) ccw
  arc A185 (-4.6999, -0.4139) -> (-4.6147, -0.3083) centre (-4.7145, -0.315) ccw
  arc A186 (-4.6999, -0.4139) -> (-5.2788, -0.6199) centre (-4.4697, -1.9771) ccw
  arc A187 (-5.2788, -0.6199) -> (-5.3267, -0.7192) centre (-5.2276, -0.7058) ccw
  arc A188 (-5.3267, -0.7192) -> (-5.2882, -0.962) centre (0, 0) ccw
  arc A189 (-5.2882, -0.962) -> (-5.212, -1.0416) centre (-5.1898, -0.9441) ccw
  arc A190 (-5.212, -1.0416) -> (-4.5978, -1.0587) centre (-4.8619, 0.4992) ccw
  arc A191 (-4.4841, -1.1328) -> (-4.5978, -1.0587) centre (-4.5811, -1.1573) ccw
  arc A192 (-4.4841, -1.1328) -> (-4.4498, -1.2611) centre (0, 0) ccw
  arc A193 (-4.5111, -1.3821) -> (-4.4498, -1.2611) centre (-4.546, -1.2883) ccw
  arc A194 (-4.5111, -1.3821) -> (-5.0345, -1.7039) centre (-3.9609, -2.8632) ccw
  arc A195 (-5.0345, -1.7039) -> (-5.0607, -1.811) centre (-4.9666, -1.7773) ccw
  arc A196 (-5.0607, -1.811) -> (-4.9726, -2.0405) centre (0, 0) ccw
  arc A197 (-4.9726, -2.0405) -> (-4.8815, -2.1025) centre (-4.8801, -2.0025) ccw
  arc A198 (-4.8815, -2.1025) -> (-4.2772, -1.9915) centre (-4.8594, -0.5226) ccw
  arc A199 (-4.1506, -2.0403) -> (-4.2772, -1.9915) centre (-4.2404, -2.0844) ccw
  arc A200 (-4.1506, -2.0403) -> (-4.0903, -2.1587) centre (0, 0) ccw
  arc A201 (-4.1252, -2.2898) -> (-4.0903, -2.1587) centre (-4.1788, -2.2053) ccw
  arc A202 (-4.1252, -2.2898) -> (-4.5702, -2.7134) centre (-3.2791, -3.6242) ccw
  arc A203 (-4.5702, -2.7134) -> (-4.5736, -2.8236) centre (-4.4885, -2.7711) ccw
  arc A204 (-4.5736, -2.8236) -> (-4.4397, -3.0297) centre (0, 0) ccw
  arc A205 (-4.4397, -3.0297) -> (-4.3377, -3.0715) centre (-4.3571, -2.9734) ccw
  arc A206 (-4.3377, -3.0715) -> (-3.7697, -2.8372) centre (-4.6446, -1.5215) ccw
  arc A207 (-3.6357, -2.8587) -> (-3.7697, -2.8372) centre (-3.7143, -2.9205) ccw
  arc A208 (-3.6357, -2.8587) -> (-3.5521, -2.9619) centre (0, 0) ccw
  arc A209 (-3.559, -3.0974) -> (-3.5521, -2.9619) centre (-3.6289, -3.026) ccw
  arc A210 (-3.559, -3.0974) -> (-3.9062, -3.6043) centre (-2.4539, -4.2268) ccw
  arc A211 (-3.9062, -3.6043) -> (-3.8866, -3.7128) centre (-3.8143, -3.6437) ccw
  arc A212 (-3.8866, -3.7128) -> (-3.7128, -3.8866) centre (0, 0) ccw
  arc A213 (-3.7128, -3.8866) -> (-3.6043, -3.9062) centre (-3.6437, -3.8143) ccw
  arc A214 (-3.6043, -3.9062) -> (-3.0974, -3.559) centre (-4.2268, -2.4539) ccw
  arc A215 (-2.9619, -3.5521) -> (-3.0974, -3.559) centre (-3.026, -3.6289) ccw
  arc A216 (-2.9619, -3.5521) -> (-2.8587, -3.6357) centre (0, 0) ccw
  arc A217 (-2.8372, -3.7697) -> (-2.8587, -3.6357) centre (-2.9205, -3.7143) ccw
  arc A218 (-2.8372, -3.7697) -> (-3.0715, -4.3377) centre (-1.5215, -4.6446) ccw
  arc A219 (-3.0715, -4.3377) -> (-3.0297, -4.4397) centre (-2.9734, -4.3571) ccw
  arc A220 (-3.0297, -4.4397) -> (-2.8236, -4.5736) centre (0, 0) ccw
  arc A221 (-2.8236, -4.5736) -> (-2.7134, -4.5702) centre (-2.7711, -4.4885) ccw
  arc A222 (-2.7134, -4.5702) -> (-2.2898, -4.1252) centre (-3.6242, -3.2791) ccw
  arc A223 (-2.1587, -4.0903) -> (-2.2898, -4.1252) centre (-2.2053, -4.1788) ccw
  arc A224 (-2.1587, -4.0903) -> (-2.0403, -4.1506) centre (0, 0) ccw
  arc A225 (-1.9915, -4.2772) -> (-2.0403, -4.1506) centre (-2.0844, -4.2404) ccw
  arc A226 (-1.9915, -4.2772) -> (-2.1025, -4.8815) centre (-0.5226, -4.8594) ccw
  arc A227 (-2.1025, -4.8815) -> (-2.0405, -4.9726) centre (-2.0025, -4.8801) ccw
  arc A228 (-2.0405, -4.9726) -> (-1.811, -5.0607) centre (0, 0) ccw
  arc A229 (-1.811, -5.0607) -> (-1.7039, -5.0345) centre (-1.7773, -4.9666) ccw
  arc A230 (-1.7039, -5.0345) -> (-1.3821, -4.5111) centre (-2.8632, -3.9609) ccw
  arc A231 (-1.2611, -4.4498) -> (-1.3821, -4.5111) centre (-1.2883, -4.546) ccw
  arc A232 (-1.2611, -4.4498) -> (-1.1328, -4.4841) centre (0, 0) ccw
  arc A233 (-1.0587, -4.5978) -> (-1.1328, -4.4841) centre (-1.1573, -4.5811) ccw
  arc A234 (-1.0587, -4.5978) -> (-1.0416, -5.212) centre (0.4992, -4.8619) ccw
  arc A235 (-1.0416, -5.212) -> (-0.962, -5.2882) centre (-0.9441, -5.1898) ccw
  arc A236 (-0.962, -5.2882) -> (-0.7192, -5.3267) centre (0, 0) ccw
  arc A237 (-0.7192, -5.3267) -> (-0.6199, -5.2788) centre (-0.7058, -5.2276) ccw
  arc A238 (-0.6199, -5.2788) -> (-0.4139, -4.6999) centre (-1.9771, -4.4697) ccw
  arc A239 (-0.3083, -4.6147) -> (-0.4139, -4.6999) centre (-0.315, -4.7145) ccw
  circle A240 centre (0, 0) radius 2.5
  dimension "d18" = 5
  constraint coincident A0.centre A4.centre
  measures "d18" diameter of A240
extrude "Extrude1" cut sketch "Cut" against normal blind 6 contours A240
named bodies: "Helical Gear"
